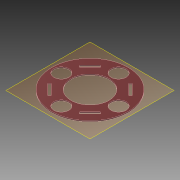
# Autodesk Inventor part: Диск_базирующий_В5
Saved by Autodesk Inventor 2021.3 (Build 253353000, 353)
## iProperties
Part Number: Диск_базирующий_В5
Checked By: Якушев
Engr Approved By: Малов
Material: По умолчанию1
Document SubType Name: Modeling
Mfg Approved By: Судаков
Designer: Смирнов
Density: 1 g/cm^3
Appearance: Каштановый
RuleStatus: InUse
AfterMaterialChange0: Материал
BeforeDocSave0: Материал
AfterAnyiPropertyChange0: Материал
Author: Смирнов
Материал: По умолчанию1
Autodesk Inventor part; units mm, degrees
ref_plane "YZ Plane" through (0, 0, 0) normal (1, 0, 0) x (0, 1, 0)
ref_plane "XZ Plane" through (0, 0, 0) normal (0, 1, 0) x (-1, 0, 0)
ref_plane "XY Plane" through (0, 0, 0) normal (0, 0, 1) x (1, 0, 0)
ref_plane "РабПлоскость1" through (0, 0, 3) normal (0, 0, 1) x (1, 0, 0)
sketch "Эскиз1" plane through (0, 0, 3) normal (0, 0, 1) x (1, 0, 0)
  circle A0 centre (0, 0) radius 101 construction
  circle A1 centre (0, 0) radius 135 projected
  line L0 (0, 0) -> (0, 153.023) construction
  circle A2 centre (0, 101) radius 26.5
  line L1 (86.9741, 51.6188) -> (51.6188, 86.9741) construction
  line L2 (51.6188, 86.9741) -> (55.8614, 91.2168) construction
  line L3 (55.8614, 91.2168) -> (91.2168, 55.8614) construction
  line L4 (91.2168, 55.8614) -> (86.9741, 51.6188) construction
  line L5 (86.9741, 51.6188) -> (55.8614, 91.2168) construction
  line L6 (51.6188, 86.9741) -> (91.2168, 55.8614) construction
  line L7 (86.9741, 50.2046) -> (50.2046, 86.9741)
  line L8 (50.2046, 86.9741) -> (55.8614, 92.631)
  line L9 (55.8614, 92.631) -> (92.631, 55.8614)
  line L10 (92.631, 55.8614) -> (86.9741, 50.2046)
  line L11 (86.9741, 50.2046) -> (55.8614, 92.631) construction
  line L12 (50.2046, 86.9741) -> (92.631, 55.8614) construction
  line L13 (-86.9741, 51.6188) -> (-91.2168, 55.8614) construction
  line L14 (-86.9741, 50.2046) -> (-92.631, 55.8614)
  circle A3 centre (-101, 0) radius 26.5
  line L15 (-91.2168, 55.8614) -> (-55.8614, 91.2168) construction
  line L16 (-86.9741, 51.6188) -> (-55.8614, 91.2168) construction
  line L17 (-51.6188, 86.9741) -> (-86.9741, 51.6188) construction
  line L18 (-51.6188, 86.9741) -> (-91.2168, 55.8614) construction
  line L19 (-86.9741, 50.2046) -> (-55.8614, 92.631) construction
  line L20 (-50.2046, 86.9741) -> (-86.9741, 50.2046)
  line L21 (-50.2046, 86.9741) -> (-92.631, 55.8614) construction
  line L22 (-55.8614, 91.2168) -> (-51.6188, 86.9741) construction
  line L23 (-55.8614, 92.631) -> (-50.2046, 86.9741)
  line L24 (-92.631, 55.8614) -> (-55.8614, 92.631)
  line L25 (-51.6188, -86.9741) -> (-55.8614, -91.2168) construction
  line L26 (-50.2046, -86.9741) -> (-55.8614, -92.631)
  circle A4 centre (0, -101) radius 26.5
  line L27 (-55.8614, -91.2168) -> (-91.2168, -55.8614) construction
  line L28 (-51.6188, -86.9741) -> (-91.2168, -55.8614) construction
  line L29 (-86.9741, -51.6188) -> (-51.6188, -86.9741) construction
  line L30 (-86.9741, -51.6188) -> (-55.8614, -91.2168) construction
  line L31 (-50.2046, -86.9741) -> (-92.631, -55.8614) construction
  line L32 (-86.9741, -50.2046) -> (-50.2046, -86.9741)
  line L33 (-86.9741, -50.2046) -> (-55.8614, -92.631) construction
  line L34 (-91.2168, -55.8614) -> (-86.9741, -51.6188) construction
  line L35 (-92.631, -55.8614) -> (-86.9741, -50.2046)
  line L36 (-55.8614, -92.631) -> (-92.631, -55.8614)
  line L37 (86.9741, -51.6188) -> (91.2168, -55.8614) construction
  line L38 (86.9741, -50.2046) -> (92.631, -55.8614)
  circle A5 centre (101, 0) radius 26.5
  line L39 (91.2168, -55.8614) -> (55.8614, -91.2168) construction
  line L40 (86.9741, -51.6188) -> (55.8614, -91.2168) construction
  line L41 (51.6188, -86.9741) -> (86.9741, -51.6188) construction
  line L42 (51.6188, -86.9741) -> (91.2168, -55.8614) construction
  line L43 (86.9741, -50.2046) -> (55.8614, -92.631) construction
  line L44 (50.2046, -86.9741) -> (86.9741, -50.2046)
  line L45 (50.2046, -86.9741) -> (92.631, -55.8614) construction
  line L46 (55.8614, -91.2168) -> (51.6188, -86.9741) construction
  line L47 (55.8614, -92.631) -> (50.2046, -86.9741)
  line L48 (92.631, -55.8614) -> (55.8614, -92.631)
  circle A6 centre (0, 0) radius 67
  point P0 (71.4178, 71.4178)
  point P1 (-71.4178, 71.4178)
  point P2 (-71.4178, -71.4178)
  point P3 (71.4178, -71.4178)
  dimension "d0" = 202
  dimension "d1" = 53
  dimension "d2" = 1
  dimension "d3" = 1
  dimension "d6" = 360
  dimension "d8" = 34
  dimension "d9" = 34
  constraints: 98 end point, 16 midpoint, 14 coincident, 5 centre point, 5 parallel, 2 perpendicular, 1 point on line, 1 vertical, 1 vertical alignment, 110 other
  measures "d1" diameter of A2
  measures "d2" distance between parallel lines of L9 L3
  measures "d3" distance between parallel lines of L2 L8
extrude "Выдавливание1" add sketch "Эскиз1" along normal blind 3
equation "\"d9\" = d8"
